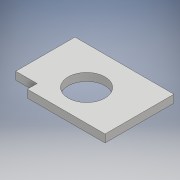
# Autodesk Inventor part: shayba kvadrat
Saved by Autodesk Inventor 2018.2 (Build 222227000, 227)
## iProperties
Created: 2026-01-20
Part Number: shayba kvadrat
Material: Типовые
Document SubType Name: Modeling
Designer: Denis
Density: 1 g/cm^3
Appearance: По умолчанию
Author: Denis
Autodesk Inventor part; units mm, degrees
ref_plane "YZ Plane" through (0, 0, 0) normal (1, 0, 0) x (0, 1, 0)
ref_plane "XZ Plane" through (0, 0, 0) normal (0, 1, 0) x (-1, 0, 0)
ref_plane "XY Plane" through (0, 0, 0) normal (0, 0, 1) x (1, 0, 0)
sketch "Эскиз1" plane through (0, 0, 0) normal (0, 0, 1) x (1, 0, 0)
  line L0 (0, 0) -> (10.2, 0)
  line L1 (10.2, 0) -> (10.2, -6.1)
  line L2 (10.2, -6.1) -> (0, -6.1)
  line L3 (0, -6.1) -> (0, 0)
  line L4 (10.2, -6.1) -> (2.2, -6.1)
  line L5 (2.2, -6.1) -> (2.2, -7.1)
  line L6 (2.2, -7.1) -> (10.2, -7.1)
  line L7 (10.2, -7.1) -> (10.2, -6.1)
  dimension "d0" = 10.2
  dimension "d1" = 6.1
  dimension "d2" = 8
  dimension "d3" = 1
  constraints: 16 end point, 4 parallel, 2 horizontal, 2 perpendicular
  measures "d0" distance of L1.end L2.end
  measures "d1" distance of L0.end L1.end
  measures "d2" distance of L6.end L5.end
  measures "d3" distance of L5.end L4.end
extrude "Выдавливание1" add sketch "Эскиз1" along normal blind 0.8
sketch "Эскиз2" plane through (0, 0, 0.8) normal (0, 0, 1) x (1, 0, 0)
  line L0 (2.2, -7.1) -> (10.2, -7.1) projected
  line L1 (10.2, -7.1) -> (10.2, -3.9)
  line L2 (10.2, -7.1) -> (10.2, 0) projected
  line L3 (10.2, -3.9) -> (5.1, -3.9)
  line L4 (0, 0) -> (0, -6.1) projected
  circle A0 centre (5.1, -3.9) radius 1.9
  dimension "d6" = 3.2
  dimension "d7" = 5.1
  dimension "d8" = 3.8
  constraints: 4 end point, 1 centre point, 1 coincident, 1 perpendicular, 1 point on line
  measures "d6" distance of L0.end L1.end
  measures "d7" distance of L1.end L3.end
  measures "d8" diameter of A0
extrude "Выдавливание2" cut sketch "Эскиз2" against normal blind 0.8
